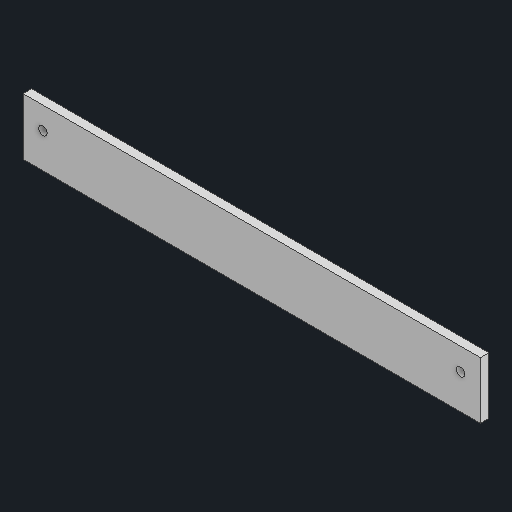
# Autodesk Inventor part: 前挡板
Saved by Autodesk Inventor 2025 (Build 290162000, 162)
## iProperties
Created: 2024-12-28
Part Number: 前挡板
Material: 常规
Document SubType Name: Modeling
Designer: HZD
Density: 1 g/cm^3
Appearance: 默认
Author: HZD
Autodesk Inventor part; units mm, degrees
ref_plane "YZ Plane" through (0, 0, 0) normal (1, 0, 0) x (0, 1, 0)
ref_plane "XZ Plane" through (0, 0, 0) normal (0, 1, 0) x (-1, 0, 0)
ref_plane "XY Plane" through (0, 0, 0) normal (0, 0, 1) x (1, 0, 0)
sketch "草图1" plane through (0, 0, 0) normal (0, 0, 1) x (1, 0, 0)
  line L0 (80.5, -10) -> (-80.5, -10)
  line L1 (-80.5, -10) -> (-80.5, 10)
  line L2 (-80.5, 10) -> (80.5, 10)
  line L3 (80.5, 10) -> (80.5, -10)
  line L4 (80.5, -10) -> (-80.5, 10) construction
  line L5 (-80.5, -10) -> (80.5, 10) construction
  point P0 (0, 0)
  dimension "d0" = 20
  dimension "d1" = 161
  constraints: 12 end point, 2 midpoint, 2 parallel, 1 horizontal, 1 perpendicular
  measures "d0" distance of L0.end L1.end
  measures "d1" distance of L1.end L2.end
extrude "拉伸1" add sketch "草图1" along normal blind 3
sketch "草图2" plane through (0, 0, 3) normal (0, 0, 1) x (1, 0, 0)
  circle A0 centre (73.5, 2.1994) radius 1.5 projected
  line L0 (80.5, 10) -> (-80.5, 10) projected
  line L1 (80.5, -10) -> (80.5, 10) projected
  line L2 (-80.5, 10) -> (80.5, 10)
  line L3 (0, 10) -> (0, -10)
  line L4 (-80.5, -10) -> (80.5, -10) projected
  circle A1 centre (-73.5, 2.1994) radius 1.5
  point P0 (0, 0)
  constraints: 4 end point, 2 midpoint, 1 centre point, 1 horizontal, 1 symmetric about line, 1 other
extrude "拉伸2" cut sketch "草图2" against normal blind 10 contours A0 | A1
